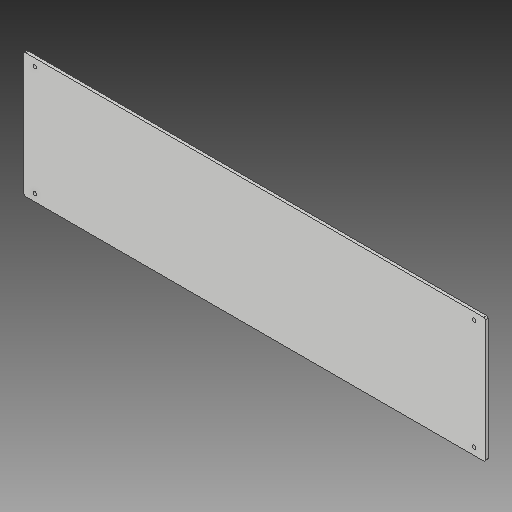
# Autodesk Inventor part: Projector Mount
Saved by Autodesk Inventor 2019 (Build 230136000, 136)
## iProperties
Created: 2020-03-17
Part Number: Projector Mount
Material: Generic
Document SubType Name: Modeling
Designer: Vijay
Density: 1 g/cm^3
Appearance: Default
Author: Vijay
Autodesk Inventor part; units mm, degrees
ref_plane "YZ Plane" through (0, 0, 0) normal (1, 0, 0) x (0, 1, 0)
ref_plane "XZ Plane" through (0, 0, 0) normal (0, 1, 0) x (-1, 0, 0)
ref_plane "XY Plane" through (0, 0, 0) normal (0, 0, 1) x (1, 0, 0)
sketch "Sketch1" plane through (0, 0, 0) normal (0, 0, 1) x (1, 0, 0)
  line L0 (-601.9604, 0.0293) -> (-602.0117, -529.9707) construction
  line L1 (28, -530) -> (28, 100) construction
  line L2 (-582.8507, 100.0274) -> (-582.9118, -529.9726) construction
  line L3 (-591.0507, 100.0282) -> (-582.8507, 100.0274) construction
  line L4 (-591.0507, 100.0282) -> (-591.1118, -529.9718) construction
  line L5 (-582.9118, -529.9726) -> (-591.1118, -529.9718) construction
  line L6 (17.1933, 99.9429) -> (17.0775, -530.057) construction
  line L7 (8.9933, 99.9444) -> (17.1933, 99.9429) construction
  line L8 (8.9933, 99.9444) -> (8.8775, -530.0555) construction
  line L9 (17.0775, -530.057) -> (8.8775, -530.0555) construction
  line L10 (12.9775, -530.0563) -> (13.0933, 99.9437) construction
  line L11 (-587.0118, -529.9722) -> (-586.9507, 100.0278) construction
  line L12 (-602.0081, -491.922) -> (28, -491.922)
  line L13 (28, -491.922) -> (28, -321.922)
  line L14 (28, -321.922) -> (-602.0081, -321.922)
  line L15 (-602.0081, -321.922) -> (-602.0081, -491.922)
  circle A0 centre (-587.0071, -481.922) radius 2.5
  circle A1 centre (-586.9926, -331.922) radius 2.5
  circle A2 centre (12.9863, -481.922) radius 2.5
  circle A3 centre (13.0139, -331.922) radius 2.5
  point P0 (0, 0)
  dimension "d0" = 170
  dimension "d1" = 5
  dimension "d2" = 5
  dimension "d3" = 5
  dimension "d4" = 5
  dimension "d5" = 10
  dimension "d6" = 10
  dimension "d7" = 10
  dimension "d8" = 10
  constraints: 14 end point, 6 point on line, 4 centre point, 4 midpoint, 2 parallel, 1 horizontal, 1 perpendicular, 1 vertical, 2 other
  measures "d0" distance between parallel lines of L12 L14
  measures "d1" diameter of A0
  measures "d2" diameter of A1
  measures "d3" diameter of A2
  measures "d4" diameter of A3
  measures "d5" distance from line of L12 A0.centre
  measures "d6" distance from line of L14 A1.centre
  measures "d7" distance from line of A2.centre L12
  measures "d8" distance from line of L14 A3.centre
extrude "Extrusion1" add sketch "Sketch1" along normal blind 4
fillet "Fillet1" radius 2 4 edges at (28, -491.922, 2) (28, -321.922, 2) (-602.0081, -321.922, 2) (-602.0081, -491.922, 2)
body "Solid1"
